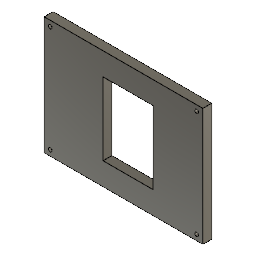
AssemblyBase (Autodesk Fusion 360 design; units mm, degrees)
Autodesk Fusion 360 part; units mm, degrees
sketch "Sketch1" plane through (0, 0, 0) normal (0, 1, 0) x (1, 0, 0)
  line L0 (0, 0) -> (350, 0)
  line L1 (350, 0) -> (350, -260)
  line L2 (350, -260) -> (0, -260)
  line L3 (0, -260) -> (0, 0)
  circle A0 centre (13.5555, -247.4318) radius 4.05
  line L4 (175, -260) -> (175, 0) construction
  line L5 (0, -130) -> (350, -130) construction
  line L6 (350, -130) -> (0, -130) construction
  circle A1 centre (336.4445, -247.4318) radius 4.05
  circle A2 centre (336.4445, -12.5682) radius 4.05
  circle A3 centre (13.5555, -12.5682) radius 4.05
  line L7 (40, -260) -> (40.238, -260)
  line L8 (130, -50) -> (240, -50)
  line L9 (130, -50) -> (130, -210)
  line L10 (130, -210) -> (240, -210)
  line L11 (240, -210) -> (240, -50)
  dimension "d1" = 350
  dimension "d2" = 260
  dimension "d3" = 8.1
  constraint horizontal L0
  constraint vertical L1
  constraint horizontal L2
  constraint vertical L3
  constraint coincident L0.start L3.end
  constraint midpoint L2 L4.start
  constraint midpoint L0 L4.end
  constraint midpoint L3 L5.start
  constraint midpoint L1 L5.end
  constraint symmetric L4 L5.start L5.end
  constraint symmetric L4 L5.end L5.start
  constraint symmetric A0 L4 A1
  constraint symmetric A0 L6 A3
  constraint symmetric L6 A1 A2
  constraint horizontal L7
  constraint coincident L2 L7.start
  constraint perpendicular L8 L9
  constraint perpendicular L4 L10
  constraint perpendicular L8 L11
  measures "d1" distance of L0.start L0.end
  measures "d2" distance of L0.start L2.end
  measures "d3" diameter of A0
extrude "Extrude1" add sketch "Sketch1" along normal blind 20
